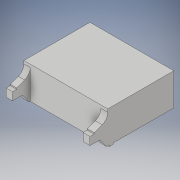
# Autodesk Inventor part: IMA Battery Case Primitive
Saved by Autodesk Inventor 2017 (Build 210142000, 142)
## iProperties
Created: 2021-05-31
Part Number: IMA Battery Case Primitive
Material: Generic
Document SubType Name: Modeling
Designer: Win240
Density: 1 g/cm^3
Appearance: Default
Author: Win240
Autodesk Inventor part; units mm, degrees
ref_plane "YZ Plane" through (0, 0, 0) normal (1, 0, 0) x (0, 1, 0)
ref_plane "XZ Plane" through (0, 0, 0) normal (0, 1, 0) x (-1, 0, 0)
ref_plane "XY Plane" through (0, 0, 0) normal (0, 0, 1) x (1, 0, 0)
sketch "Sketch1" plane through (0, 0, 0) normal (0, 0, 1) x (1, 0, 0)
  line L0 (-212.5, -81.5) -> (212.5, -81.5)
  line L1 (212.5, -81.5) -> (212.5, 81.5)
  line L2 (212.5, 81.5) -> (-212.5, 81.5)
  line L3 (-212.5, 81.5) -> (-212.5, -81.5)
  line L4 (-212.5, -81.5) -> (212.5, 81.5) construction
  line L5 (212.5, -81.5) -> (-212.5, 81.5) construction
  point P0 (0, 0)
  dimension "d0" = 163
  dimension "d1" = 425
  constraints: 12 end point, 2 midpoint, 2 parallel, 1 horizontal, 1 perpendicular
  measures "d0" distance of L0.end L1.end
  measures "d1" distance of L1.end L2.end
extrude "Extrusion1" add sketch "Sketch1" against normal blind 335
sketch "Sketch2" plane through (-212.5, -81.5, 0) normal (0, -1, 0) x (1, 0, 0)
  line L0 (0, 0) -> (425, 0) construction
  line L1 (425, -8) -> (409.5, -8)
  line L2 (409.5, -8) -> (409.5, -28)
  line L3 (409.5, -28) -> (425, -28)
  line L4 (425, -28) -> (425, -8)
  line L5 (20, -10) -> (0, -10)
  line L6 (0, -10) -> (0, -25.5)
  line L7 (0, -25.5) -> (20, -25.5)
  line L8 (20, -25.5) -> (20, -10)
  line L9 (0, -10) -> (0, 0) construction
  line L10 (425, -8) -> (425, 0) construction
  point P0 (212.5, 0)
  dimension "d4" = 8
  dimension "d5" = 10
  dimension "d6" = 15.5
  dimension "d7" = 20
  dimension "d8" = 15.5
  dimension "d9" = 20
  constraints: 20 end point, 4 parallel, 2 horizontal, 2 perpendicular, 2 vertical
  measures "d4" distance between parallel lines of L0 L1
  measures "d5" distance between parallel lines of L5 L0
  measures "d6" distance of L1.start L1.end
  measures "d7" distance of L5.start L5.end
  measures "d8" distance of L7.end L5.start
  measures "d9" distance of L3.end L1.start
extrude "Extrusion2" add sketch "Sketch2" along normal blind 6
sketch "Sketch3" plane through (212.5, -81.5, 0) normal (1, 0, 0) x (0, 0, -1)
  line L0 (0, 0) -> (0, 163) projected
  line L1 (0, 0) -> (-5, 0)
  line L2 (-5, 0) -> (-40, 47)
  line L3 (-40, 47) -> (-90, 47)
  line L4 (-90, 47) -> (-90, 87)
  line L5 (-90, 87) -> (-69, 87)
  line L6 (-69, 93) -> (-28.2057, 107.7805)
  line L7 (-69, 87) -> (-69, 93)
  arc A0 (-28.2057, 107.7805) -> (0, 148) centre (-42.778, 148) ccw
  line L8 (-28.2057, 107.7805) -> (0, 118) construction
  arc A1 (-37.8496, 44.1124) -> (-43.6003, 47) centre (-43.6003, 39.8299) ccw
  dimension "d12" = 5
  dimension "d13" = 47
  dimension "d14" = 35
  dimension "d15" = 40
  dimension "d16" = 90
  dimension "d17" = 118
  dimension "d18" = 93
  dimension "d19" = 69
  dimension "d22" = 15
  dimension "d23" = 55
  constraints: 16 end point, 5 tangent, 4 point on circle, 4 point on line, 3 horizontal, 2 centre point, 2 vertical
  measures "d12" distance of L0.start L1.end
  measures "d13" distance between parallel lines of L1 L3
  measures "d14" horizontal distance of L1.end L2.end
  measures "d15" distance of L3.end L4.end
  measures "d16" distance between parallel lines of L0 L4
  measures "d17" distance from line of L8.end L1
  measures "d18" distance from line of L1 L6.start
  measures "d19" distance between parallel lines of L0 L7
  measures "d22" distance of A0.end L0.end
  measures "d23" distance of L1.end A1.start
extrude "Extrusion3" add sketch "Sketch3" against normal blind 35
sketch "Sketch4" plane through (-212.5, -81.5, 0) normal (-1, 0, 0) x (0, 0, 1)
  line L0 (0, 0) -> (0, 148) projected
  line L1 (0, 0) -> (5, 0) projected
  line L2 (5, 0) -> (37.8496, 44.1124) projected
  arc A0 (43.6003, 47) -> (37.8496, 44.1124) centre (43.6003, 39.8299) ccw projected
  line L3 (43.6003, 47) -> (90, 47) projected
  line L4 (90, 47) -> (90, 87) projected
  line L5 (90, 87) -> (69, 87) projected
  line L6 (69, 87) -> (69, 93) projected
  line L7 (69, 93) -> (28.2057, 107.7805) projected
  arc A1 (0, 148) -> (28.2057, 107.7805) centre (42.778, 148) ccw projected
  point P0 (0, 81.5)
extrude "Extrusion4" add sketch "Sketch4" against normal blind 32
body "Solid1"
